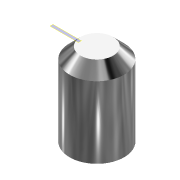
# Autodesk Inventor part: objectivelens
Saved by Autodesk Inventor 2019.4 (Build 234330000, 330)
## iProperties
Created: 2020-09-02
Part Number: objectivelens
Material: Generic
Document SubType Name: Modeling
Designer: diederichbenedict
Density: 1 g/cm^3
Appearance: Chrome - Polished
Author: diederichbenedict
Autodesk Inventor part; units mm, degrees
ref_plane "YZ Plane" through (0, 0, 0) normal (1, 0, 0) x (0, 1, 0)
ref_plane "XZ Plane" through (0, 0, 0) normal (0, 1, 0) x (-1, 0, 0)
ref_plane "XY Plane" through (0, 0, 0) normal (0, 0, 1) x (1, 0, 0)
ref_plane "Work Plane1" through (54.8357, -44, -44.5) normal (0, -1, 0) x (0, 0, -1)
sketch "Sketch1" plane through (54.8357, -44, -44.5) normal (0, -1, 0) x (0, 0, -1)
  circle A0 centre (8.0663, 17.2551) radius 49.5395
  point P0 (-44.5, -54.8357)
  constraints: 1 centre point
extrude "Extrusion1" add sketch "Sketch1" along normal blind 150
chamfer "Chamfer1" distance 20 angle 45 1 edges at (72.0908, -44, -3.0268)
body "Solid1"
